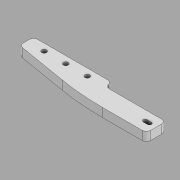
# Autodesk Inventor part: 102.001.02_Anbindung_Vereinzelung
Saved by Autodesk Inventor 2021 (Build 250183000, 183)
## iProperties
Created: 2021-11-26
Part Number: 102.001.02_Anbindung_Vereinzelung
Material: Generisch
Document SubType Name: Modeling
Designer: Oliver Ungerer
Density: 1 g/cm^3
Appearance: Vorgabe
Author: Oliver Ungerer
Autodesk Inventor part; units mm, degrees
ref_plane "YZ Plane" through (0, 0, 0) normal (1, 0, 0) x (0, 1, 0)
ref_plane "XZ Plane" through (0, 0, 0) normal (0, 1, 0) x (-1, 0, 0)
ref_plane "XY Plane" through (0, 0, 0) normal (0, 0, 1) x (1, 0, 0)
sketch "Skizze6" plane through (0, 0, 0) normal (0, 1, 0) x (-1, 0, 0)
  line L0 (69, 0) -> (158, 0)
  line L1 (158, 0) -> (158, 16)
  line L2 (0, 30) -> (0, 8)
  line L3 (0, 8) -> (69, 8)
  line L4 (69, 8) -> (69, 0)
  line L5 (0, 30) -> (75, 30)
  line L6 (75, 30) -> (158, 16)
  point P0 (0, 0)
  dimension "d34" = 89
  dimension "d35" = 22
  dimension "d36" = 30
  dimension "d37" = 158
  dimension "d38" = 75
  dimension "d41" = 16
  constraints: 14 end point, 3 perpendicular, 2 horizontal, 2 point on line, 1 parallel
  measures "d34" distance between parallel lines of L4 L1
  measures "d35" distance from line of L2.start L3
  measures "d36" distance from line of L5 point (0, 0)
  measures "d37" distance from line of point (0, 0) L1
  measures "d38" distance of L2.start L5.end
  measures "d41" distance of L0.end L1.end
extrude "Extrusion2" add sketch "Skizze6" along normal blind 10
sketch "Skizze7" plane through (0, 10, 0) normal (0, 1, 0) x (1, 0, 0)
  line L0 (-69, 0) -> (-158, 0) projected
  line L1 (-158, 0) -> (-158, -16) projected
  point P0 (0, 0)
  point P1 (-138, -8)
  point P2 (-113.5, -8)
  point P3 (-89, -8)
  point P4 (-138.2626, -14.3361)
  dimension "d42" = 8
  dimension "d43" = 20
  dimension "d44" = 24.5
  dimension "d45" = 24.5
  measures "d42" distance from line of point (-138, -8) L0
  measures "d43" distance from line of point (-138, -8) L1
  measures "d44" distance of point (-113.5, -8) point (-138, -8)
  measures "d45" distance of point (-89, -8) point (-113.5, -8)
hole "Bohrung5" at (-113.5, 10, 8) at (-89, 10, 8) at (-138, 10, 8) direction (0, -1, 0) diameter 5.5 end through all
sketch "Skizze8" plane through (0, 0, 0) normal (0, -1, 0) x (1, 0, 0)
  arc A0 (-12.5, 21.25) -> (-12.5, 16.75) centre (-12.5, 19) ccw
  line L0 (-75, 30) -> (0, 30) projected
  arc A1 (-7.5, 16.75) -> (-7.5, 21.25) centre (-7.5, 19) ccw
  line L1 (-7.5, 16.75) -> (-12.5, 16.75)
  line L2 (-7.5, 21.25) -> (-12.5, 21.25)
  line L3 (0, 30) -> (0, 8) projected
  line L4 (-158, 0) -> (-158, 16) projected
  point P0 (0, 0)
  dimension "d53" = 4.5
  dimension "d54" = 11
  dimension "d55" = 4.5
  dimension "d56" = 5
  dimension "d58" = 145.5
  constraints: 4 end point, 4 point on circle, 4 tangent, 2 centre point, 1 parallel
  measures "d53" diameter of A0
  measures "d54" distance from line of A0.centre L0
  measures "d55" diameter of A1
  measures "d56" distance of A1.centre A0.centre
  measures "d58" distance from line of L4 A0.centre
extrude "Extrusion3" cut sketch "Skizze8" against normal through all
fillet "Rundung1" radius 5 6 edges at (-69, 5, 8) (-69, 5, 0) (0, 5, 8) (0, 5, 30) (-158, 5, 16) (-158, 5, 0)
fillet "Rundung2" radius 300 1 edges at (-75, 5, 30)
